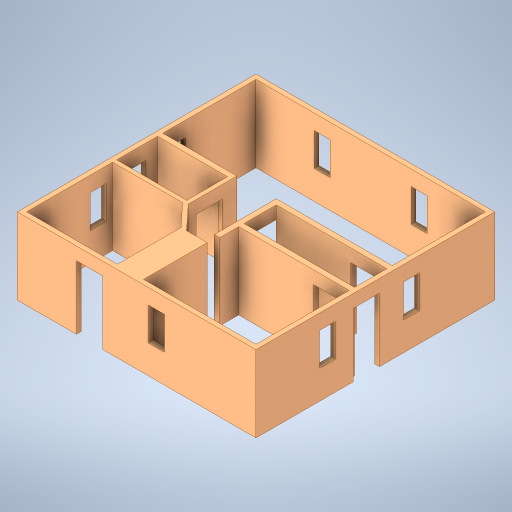
# Autodesk Inventor part: Existing_Kitchen_And_Dining_Room
Saved by Autodesk Inventor 2024 (Build 280153000, 153)
## iProperties
Created: 2023-04-15
Part Number: Existing_Kitchen_And_Dining_Room
Material: Generic
Document SubType Name: Modeling
Designer: Tom
Density: 1 g/cm^3
Appearance: Cherry - Natural Low Gloss
Author: Tom
Autodesk Inventor part; units mm, degrees
ref_plane "YZ Plane" through (0, 0, 0) normal (1, 0, 0) x (0, 1, 0)
ref_plane "XZ Plane" through (0, 0, 0) normal (0, 1, 0) x (-1, 0, 0)
ref_plane "XY Plane" through (0, 0, 0) normal (0, 0, 1) x (1, 0, 0)
sketch "Sketch1" plane through (0, 0, 0) normal (0, 1, 0) x (-1, 0, 0)
  line L0 (149.225, -7464.425) -> (149.225, 149.225)
  line L1 (149.225, 149.225) -> (-7464.425, 149.225)
  line L2 (-7464.425, 149.225) -> (-7464.425, -7464.425)
  line L3 (-7464.425, -7464.425) -> (149.225, -7464.425)
  line L4 (149.225, -2874.0552) -> (149.225, -3026.323)
  line L5 (0, 0) -> (0, -7315.2)
  line L6 (0, -7315.2) -> (-7315.2, -7315.2)
  line L7 (-7315.2, -7315.2) -> (-7315.2, 0)
  line L8 (-7315.2, 0) -> (0, 0)
  line L9 (0, -2740.8208) -> (-2233.2614, -2740.8208)
  line L10 (-2233.2614, -2740.8208) -> (-2893.0886, -2030.2376)
  line L11 (-2893.0886, -2030.2376) -> (-2893.0886, 0)
  line L12 (0, -2870.8829) -> (-2233.2614, -2870.8829)
  line L13 (-2233.2614, -2870.8829) -> (-2233.2614, -4171.95)
  line L14 (-2233.2614, -4171.95) -> (0, -4171.95)
  line L15 (0, -4343.4) -> (-2363.3235, -4343.4)
  line L16 (-2363.3235, -4343.4) -> (-2363.3235, -2791.8949)
  line L17 (-2363.3235, -2791.8949) -> (-3070.5767, -2030.2376)
  line L18 (-3070.5767, -2030.2376) -> (-3730.4039, -2030.2376)
  line L19 (-3730.4039, -2030.2376) -> (-3730.4039, 0)
  line L20 (-7315.2, -3143.25) -> (-3790.8343, -3143.25)
  line L21 (-3790.8343, -3143.25) -> (-3790.8343, -4171.95)
  line L22 (-3619.3843, -4343.4) -> (-3619.3843, -2360.2792)
  line L23 (-3790.8343, -2971.8) -> (-7315.2, -2971.8)
  line L24 (-3619.3843, -4343.4) -> (-7315.2, -4343.4)
  line L25 (-7315.2, -4171.95) -> (-3790.8343, -4171.95)
  line L26 (-3790.8343, -2971.8) -> (-3790.8343, -2360.2792)
  line L27 (-3790.8343, -2360.2792) -> (-3619.3843, -2360.2792)
  dimension "d145" = 7315.2
  dimension "d146" = 149.225
  dimension "d147" = 2971.8
  dimension "d148" = 171.45
  dimension "d149" = 171.45
  dimension "d150" = 171.45
  dimension "d151" = 2971.8
  constraints: 56 end point, 12 perpendicular, 10 point on line, 6 horizontal, 4 collinear, 3 parallel, 1 coincident, 3 other
  measures "d145" distance of L5.end L6.end
  measures "d146" distance between parallel lines of L3 L6
  measures "d147" distance between parallel lines of L6 L24
  measures "d148" distance between parallel lines of L25 L24
  measures "d149" distance between parallel lines of L22 L21
  measures "d150" distance between parallel lines of L20 L23
  measures "d151" distance between parallel lines of L8 L23
extrude "Extrusion1" add sketch "Sketch1" along normal blind 2438.4 contours L3 L2 L1 L0 | L5 L12 L13 L14 L15 L16 L17 L18 L19 L8 L11 L10 L9 | L23 L26 L27 L22 L24 L7 L25 L21 L20
sketch "Sketch2" plane through (-149.225, 0, -7464.425) normal (-1, 0, 0) x (0, 0, 1)
  line L0 (4933.1542, 1955.8) -> (5441.1542, 1955.8)
  line L1 (5441.1542, 1955.8) -> (5441.1542, 914.4)
  line L2 (5441.1542, 914.4) -> (4933.1542, 914.4)
  line L3 (4933.1542, 914.4) -> (4933.1542, 1955.8)
  line L4 (0, 0) -> (7613.65, 0) projected
  line L5 (2911.475, 1955.8) -> (2403.475, 1955.8)
  line L6 (2403.475, 1955.8) -> (2403.475, 914.4)
  line L7 (2403.475, 914.4) -> (2911.475, 914.4)
  line L8 (2911.475, 914.4) -> (2911.475, 1955.8)
  line L9 (3660.775, 1955.8) -> (4702.175, 1955.8)
  line L10 (4702.175, 1955.8) -> (4702.175, 914.4)
  line L11 (4702.175, 914.4) -> (3660.775, 914.4)
  line L12 (3660.775, 914.4) -> (3660.775, 1955.8)
  point P0 (7464.425, 0)
  point P1 (4723.6042, 2438.4)
  point P2 (3121.025, 2438.4)
  point P3 (3292.475, 2438.4)
  dimension "d63" = 914.4
  dimension "d64" = 209.55
  dimension "d65" = 508
  dimension "d66" = 1041.4
  dimension "d67" = 209.55
  dimension "d68" = 508
  dimension "d69" = 1041.4
  dimension "d70" = 914.4
  dimension "d71" = 914.4
  dimension "d72" = 1041.4
  dimension "d73" = 1041.4
  dimension "d74" = 368.3
  constraints: 24 end point, 6 parallel, 3 horizontal, 3 perpendicular
  measures "d63" distance between parallel lines of L4 L2
  measures "d64" distance from line of L3 point (4723.604, 2438.4)
  measures "d65" distance of L0.start L0.end
  measures "d66" distance of L0.end L1.end
  measures "d67" distance from line of L8 point (3121.025, 2438.4)
  measures "d68" distance of L5.start L5.end
  measures "d69" distance of L5.end L6.end
  measures "d70" distance between parallel lines of L4 L7
  measures "d71" distance between parallel lines of L4 L11
  measures "d72" distance of L11.end L9.start
  measures "d73" distance of L9.start L9.end
  measures "d74" distance from line of L12 point (3292.475, 2438.4)
extrude "Extrusion2" cut sketch "Sketch2" against normal up to surface (149.225 mm away)
sketch "Sketch3" plane through (7464.425, 0, -7464.425) normal (0, 0, -1) x (-1, 0, 0)
  line L0 (5099.05, 1955.8) -> (5607.05, 1955.8)
  line L1 (5607.05, 1955.8) -> (5607.05, 914.4)
  line L2 (5607.05, 914.4) -> (5099.05, 914.4)
  line L3 (5099.05, 914.4) -> (5099.05, 1955.8)
  line L4 (0, 0) -> (7613.65, 0) projected
  line L5 (7464.425, 0) -> (7464.425, 2438.4) projected
  line L6 (2006.6, 1955.8) -> (2514.6, 1955.8)
  line L7 (2514.6, 1955.8) -> (2514.6, 914.4)
  line L8 (2514.6, 914.4) -> (2006.6, 914.4)
  line L9 (2006.6, 914.4) -> (2006.6, 1955.8)
  line L10 (149.225, 0) -> (149.225, 2438.4) projected
  dimension "d78" = 1041.4
  dimension "d79" = 508
  dimension "d80" = 2365.375
  dimension "d81" = 2365.375
  dimension "d82" = 1041.4
  dimension "d83" = 508
  dimension "d84" = 914.4
  dimension "d85" = 914.4
  constraints: 16 end point, 4 parallel, 2 horizontal, 2 perpendicular
  measures "d78" distance of L0.end L1.end
  measures "d79" distance of L0.start L0.end
  measures "d80" distance between parallel lines of L5 L3
  measures "d81" distance between parallel lines of L10 L7
  measures "d82" distance of L6.end L7.end
  measures "d83" distance of L6.start L6.end
  measures "d84" distance between parallel lines of L4 L8
  measures "d85" distance between parallel lines of L4 L2
extrude "Extrusion3" cut sketch "Sketch3" against normal up to surface (149.225 mm away)
sketch "Sketch4" plane through (7464.425, 0, 149.225) normal (1, 0, 0) x (0, 0, -1)
  line L0 (4702.175, 1955.8) -> (5210.175, 1955.8)
  line L1 (5210.175, 1955.8) -> (5210.175, 914.4)
  line L2 (5210.175, 914.4) -> (4702.175, 914.4)
  line L3 (4702.175, 914.4) -> (4702.175, 1955.8)
  line L4 (0, 0) -> (7613.65, 0) projected
  line L5 (2533.65, 1955.8) -> (2025.65, 1955.8)
  line L6 (2025.65, 1955.8) -> (2025.65, 914.4)
  line L7 (2025.65, 914.4) -> (2533.65, 914.4)
  line L8 (2533.65, 914.4) -> (2533.65, 1955.8)
  line L9 (0, 0) -> (0, 2438.4) projected
  line L10 (4321.175, 0) -> (3292.475, 0) projected
  line L11 (3936.8412, 0) -> (3098.6412, 0)
  line L12 (3098.6412, 0) -> (3098.6412, 2032)
  line L13 (3098.6412, 2032) -> (3936.8412, 2032)
  line L14 (3936.8412, 2032) -> (3936.8412, 0)
  point P0 (149.225, 0)
  point P1 (4492.625, 2438.4)
  point P2 (4321.175, 2438.4)
  dimension "d88" = 209.55
  dimension "d89" = 508
  dimension "d90" = 1041.4
  dimension "d91" = 914.4
  dimension "d92" = 508
  dimension "d94" = 1041.4
  dimension "d97" = 2533.65
  dimension "d98" = 914.4
  dimension "d110" = 838.2
  dimension "d112" = 384.3338
  dimension "d113" = 2032
  constraints: 24 end point, 6 parallel, 3 horizontal, 3 perpendicular, 1 point on line
  measures "d88" distance from line of point (4492.625, 2438.4) L3
  measures "d89" distance of L0.start L0.end
  measures "d90" distance of L0.end L1.end
  measures "d91" distance between parallel lines of L4 L2
  measures "d92" distance of L5.start L5.end
  measures "d94" distance of L7.end L5.start
  measures "d97" distance between parallel lines of L9 L8
  measures "d98" distance between parallel lines of L4 L7
  measures "d110" distance of L12.end L13.end
  measures "d112" distance from line of point (4321.175, 2438.4) L14
  measures "d113" distance of L11.end L12.end
extrude "Extrusion4" cut sketch "Sketch4" against normal up to surface (149.225 mm away)
sketch "Sketch5" plane through (-149.225, 0, 149.225) normal (0, 0, 1) x (1, 0, 0)
  line L0 (0, 0) -> (7613.65, 0) projected
  line L1 (2724.15, 0) -> (1885.95, 0)
  line L2 (1885.95, 0) -> (1885.95, 2032)
  line L3 (1885.95, 2032) -> (2724.15, 2032)
  line L4 (2724.15, 2032) -> (2724.15, 0)
  line L5 (0, 0) -> (0, 2438.4) projected
  line L6 (4184.4289, 1955.8) -> (4692.4289, 1955.8)
  line L7 (4692.4289, 1955.8) -> (4692.4289, 914.4)
  line L8 (4692.4289, 914.4) -> (4184.4289, 914.4)
  line L9 (4184.4289, 914.4) -> (4184.4289, 1955.8)
  point P0 (149.225, 0)
  point P1 (3879.6289, 2438.4)
  point P2 (1885.95, 0)
  point P3 (149.225, 2438.4)
  dimension "d102" = 838.2
  dimension "d103" = 2032
  dimension "d104" = 304.8
  dimension "d105" = 508
  dimension "d106" = 914.4
  dimension "d107" = 1041.4
  dimension "d114" = 1736.725
  constraints: 16 end point, 4 parallel, 2 horizontal, 2 perpendicular, 1 point on line
  measures "d102" distance between parallel lines of L4 L2
  measures "d103" distance between parallel lines of L0 L3
  measures "d104" distance from line of point (3879.629, 2438.4) L9
  measures "d105" distance of L6.start L6.end
  measures "d106" distance between parallel lines of L0 L8
  measures "d107" distance of L6.end L7.end
  measures "d114" distance from line of L2 point (149.225, 2438.4)
extrude "Extrusion5" cut sketch "Sketch5" against normal up to surface (149.225 mm away)
sketch "Sketch6" plane through (2893.0886, 0, -2030.2376) normal (-0.7327935, 0, 0.6804511) x (0.6804511, 0, 0.7327935)
  line L0 (120.7719, 0) -> (-918.6168, 0) projected
  line L1 (-55.2909, 0) -> (-893.4909, 0)
  line L2 (-893.4909, 0) -> (-893.4909, 2032)
  line L3 (-893.4909, 2032) -> (-55.2909, 2032)
  line L4 (-55.2909, 2032) -> (-55.2909, 0)
  line L5 (-969.6909, 0) -> (-969.6909, 2438.4) projected
  point P0 (-480.8604, 0)
  point P1 (-893.4909, 0)
  dimension "d115" = 838.2
  dimension "d116" = 76.2
  dimension "d117" = 2032
  constraints: 8 end point, 2 parallel, 1 horizontal, 1 perpendicular, 1 point on line
  measures "d115" distance of L2.end L3.end
  measures "d116" distance between parallel lines of L5 L2
  measures "d117" distance of L3.end L1.start
extrude "Extrusion6" cut sketch "Sketch6" against normal up to surface (130.0621 mm away)
sketch "Sketch7" plane through (2363.3235, 0, -2791.8949) normal (1, 0, 0) x (0, 0, -1)
  line L0 (1084.6213, 0) -> (246.4213, 0)
  line L1 (246.4213, 0) -> (246.4213, 2032)
  line L2 (246.4213, 2032) -> (1084.6213, 2032)
  line L3 (1084.6213, 2032) -> (1084.6213, 0)
  line L4 (0, 0) -> (1551.5051, 0) projected
  line L5 (1551.5051, 0) -> (1551.5051, 2438.4) projected
  point P0 (-2791.8949, 0)
  dimension "d120" = 838.2
  dimension "d121" = 466.8838
  dimension "d122" = 2032
  constraints: 8 end point, 2 parallel, 1 collinear, 1 horizontal, 1 perpendicular
  measures "d120" distance of L1.end L2.end
  measures "d121" distance between parallel lines of L5 L3
  measures "d122" distance of L2.end L0.start
extrude "Extrusion7" cut sketch "Sketch7" against normal up to surface (130.0621 mm away)
sketch "Sketch8" plane through (3790.8343, 0, -3143.25) normal (1, 0, 0) x (0, 0, -1)
  line L0 (1200.15, 0) -> (-782.9708, 0) projected
  line L1 (1228.8837, 0) -> (390.6837, 0)
  line L2 (390.6837, 0) -> (390.6837, 2032)
  line L3 (390.6837, 2032) -> (1228.8837, 2032)
  line L4 (1228.8837, 2032) -> (1228.8837, 0)
  point P0 (-3143.25, 0)
  point P1 (0, 2438.4)
  point P2 (390.6837, 0)
  dimension "d125" = 838.2
  dimension "d126" = 390.6837
  dimension "d127" = 2032
  constraints: 8 end point, 2 parallel, 1 horizontal, 1 perpendicular, 1 point on line
  measures "d125" distance of L2.end L3.end
  measures "d126" distance from line of point (0, 2438.4) L2
  measures "d127" distance of L3.end L1.start
extrude "Extrusion8" cut sketch "Sketch8" against normal up to surface (171.45 mm away)
sketch "Sketch9" plane through (3619.3843, 0, -2971.8) normal (0, 0, 1) x (1, 0, 0)
  line L0 (0, 0) -> (3695.8157, 0) projected
  line L1 (3391.0157, 0) -> (2552.8157, 0)
  line L2 (2552.8157, 0) -> (2552.8157, 2032)
  line L3 (2552.8157, 2032) -> (3391.0157, 2032)
  line L4 (3391.0157, 2032) -> (3391.0157, 0)
  point P0 (-3619.3843, 0)
  point P1 (3695.8157, 2438.4)
  point P2 (2552.8157, 0)
  dimension "d130" = 304.8
  dimension "d132" = 2032
  dimension "d133" = 838.2
  constraints: 8 end point, 2 parallel, 1 horizontal, 1 perpendicular, 1 point on line
  measures "d130" distance from line of point (3695.816, 2438.4) L4
  measures "d132" distance of L1.end L2.end
  measures "d133" distance between parallel lines of L2 L4
extrude "Extrusion9" cut sketch "Sketch9" against normal up to surface (171.45 mm away)
sketch "Sketch10" plane through (7315.2, 0, -4343.4) normal (0, 0, -1) x (-1, 0, 0)
  line L0 (0, 0) -> (3695.8157, 0) projected
  line L1 (304.8, 0) -> (1143, 0)
  line L2 (1143, 0) -> (1143, 2032)
  line L3 (1143, 2032) -> (304.8, 2032)
  line L4 (304.8, 2032) -> (304.8, 0)
  point P0 (7315.2, 0)
  point P1 (0, 2438.4)
  point P2 (1143, 0)
  dimension "d136" = 2032
  dimension "d137" = 304.8
  dimension "d138" = 838.2
  constraints: 8 end point, 2 parallel, 1 horizontal, 1 perpendicular, 1 point on line
  measures "d136" distance of L1.end L2.end
  measures "d137" distance from line of point (0, 2438.4) L4
  measures "d138" distance of L2.end L3.end
extrude "Extrusion10" cut sketch "Sketch10" against normal up to surface (171.45 mm away)
body "Solid1"
